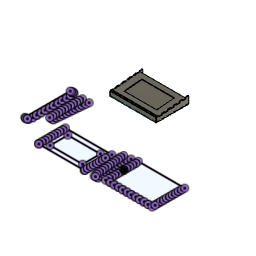
lazerskurður v8 (Autodesk Fusion 360 design; units mm, degrees)
Autodesk Fusion 360 part; units mm, degrees
sketch "Sketch1" plane through (0, 0, 0) normal (0, 0, 1) x (1, 0, 0)
  line L0 (0, 0) -> (314, 0)
  line L1 (314, 0) -> (314, 220)
  line L2 (314, 220) -> (0, 220)
  line L3 (0, 220) -> (0, 0)
  dimension "d8" = 314
  dimension "d9" = 220
  constraint horizontal L0
  constraint vertical L1
  constraint horizontal L2
  constraint vertical L3
  constraint coincident L0.start L3.end
  measures "d8" distance of L0.start L0.end
  measures "d9" distance of L0.start L2.end
extrude "Extrude1" add sketch "Sketch1" along normal blind 4 makes body 1
sketch "Sketch2" plane through (0, 0, 0) normal (0, -1, 0) x (1, 0, 0)
  line L0 (0, 0) -> (314, 0)
  line L1 (314, 0) -> (314, 4)
  line L2 (314, 4) -> (0, 4)
  line L3 (0, 4) -> (0, 0)
sketch "Sketch3" plane through (0, 0, 0) normal (-1, 0, 0) x (0, -1, 0)
  line L0 (-220, 0) -> (0, 0)
  line L1 (0, 0) -> (0, 4)
  line L2 (0, 4) -> (-220, 4)
  line L3 (-220, 4) -> (-220, 0)
  line L4 (-200, 0) -> (-180, 0)
  line L5 (-180, 0) -> (-180, 4)
  line L6 (-180, 4) -> (-200, 4)
  line L7 (-200, 4) -> (-200, 0)
  dimension "d12" = 20
  dimension "d13" = 20
  constraint horizontal L4
  constraint vertical L5
  constraint horizontal L6
  constraint vertical L7
  constraint coincident L2 L5.end
  constraint coincident L0 L4.start
  measures "d12" distance of L5.end L6.end
  measures "d13" distance of L3 L7
extrude "Extrude2" cut sketch "Sketch3" against normal blind 4 contours L0 L2 L4 L5 L6 L7 bodies 1
pattern_linear "R-Pattern1" count 5 spacing 40 along (0, -1, 0) of "Extrude2"
sketch "Sketch4" plane through (0, 0, 0) normal (1, 0, 0) x (0, 1, 0)
  line L0 (220, 0) -> (220, 50)
  line L1 (0, 0) -> (0, 30)
  line L2 (0, 30) -> (220, 50)
  line L3 (0, 30) -> (0, 0)
  line L4 (220, 0) -> (0, 0)
  dimension "d20" = 50
  dimension "d21" = 30
  constraint vertical L0
  constraint coincident L1.start L3.end
  constraint vertical L1
  constraint perpendicular L3 L4
  measures "d20" distance of L0.start L0.end
  measures "d21" distance of L1.start L1.end
extrude "Extrude3" add sketch "Sketch4" along normal blind 4 separate body makes body 2
combine "Combine1" operation cut target body 2 tool bodies 1 keep tools
sketch "Sketch5" plane through (0, -2.7049, 29.7541) normal (0, -0.090536, 0.995893) x (1, 0, 0)
  line L0 (0, 223.6233) -> (0, 2.7161)
  line L1 (0, 2.7161) -> (4, 2.7161)
  line L2 (4, 2.7161) -> (4, 223.6233)
  line L3 (4, 223.6233) -> (0, 223.6233)
  line L4 (0, 203.5408) -> (4, 203.5408)
  line L5 (4, 203.5408) -> (4, 183.4583)
  line L6 (4, 183.4583) -> (0, 183.4583)
  line L7 (0, 183.4583) -> (0, 203.5408)
  dimension "d27" = 20.0825
  dimension "d28" = 20.0825
  constraint horizontal L4
  constraint vertical L5
  constraint horizontal L6
  constraint vertical L7
  constraint coincident L2 L5.end
  constraint coincident L0 L4.start
  measures "d27" distance of L4.start L6.end
  measures "d28" distance of L3 L4
extrude "Extrude4" cut sketch "Sketch5" against normal blind 8 contours L0 L2 L4 L5 L6 L7 bodies 2
pattern_linear "R-Pattern2" count 5 spacing 40.1649 along (0, -0.995893, -0.090536) of "Extrude4"
sketch "Sketch6" plane through (0, -1.9806, 21.787) normal (0, -0.090536, 0.995893) x (1, 0, 0)
  line L0 (0, 183.4583) -> (4, 183.4583)
  line L1 (4, 183.4583) -> (4, 203.5408)
  line L2 (4, 203.5408) -> (0, 203.5408)
  line L3 (0, 203.5408) -> (0, 183.4583)
  line L4 (0, 220) -> (310, 220)
  line L5 (310, 220) -> (310, 0)
  line L6 (310, 0) -> (0, 0)
  line L7 (0, 220) -> (0, 0)
  constraint perpendicular L1 L4
  constraint perpendicular L2 L5
  constraint coincident L6.end L7.end
  constraint perpendicular L5 L6
  constraint perpendicular L6 L7
combine "Combine2" operation cut target body 1 tool bodies 2 keep tools
sketch "Sketch7" plane through (0, 0, 0) normal (0, -1, 0) x (1, 0, 0)
  line L0 (28.5455, 4) -> (57.0909, 4)
  line L1 (57.0909, 4) -> (57.0909, 0)
  line L2 (57.0909, 0) -> (28.5455, 0)
  line L3 (28.5455, 0) -> (28.5455, 4)
  line L4 (0, 4) -> (0, 0)
  dimension "d42" = 28.5455
  dimension "d43" = 28.5455
  constraint horizontal L0
  constraint vertical L1
  constraint horizontal L2
  constraint vertical L3
  measures "d42" distance of L0.start L0.end
  measures "d43" distance of L3 L4
extrude "Extrude7" cut sketch "Sketch7" against normal blind 4 bodies 1
pattern_linear "R-Pattern3" count 5 spacing 57.0909 along (1, 0, 0) of "Extrude7"
sketch "Sketch11" plane through (0, 0, 0) normal (0, -1, 0) x (1, 0, 0)
  line L0 (0, 4) -> (4, 4)
  line L1 (4, 4) -> (4, 30)
  line L2 (4, 30) -> (0, 30)
  line L3 (0, 30) -> (0, 4)
  line L4 (0, 12.6667) -> (4, 12.6667)
  line L5 (4, 12.6667) -> (4, 21.3333)
  line L6 (4, 21.3333) -> (0, 21.3333)
  line L7 (0, 21.3333) -> (0, 12.6667)
  dimension "d56" = 8.6667
  dimension "d57" = 8.6667
  constraint horizontal L4
  constraint vertical L5
  constraint horizontal L6
  constraint vertical L7
  constraint coincident L1 L5.end
  constraint coincident L3 L4.start
  measures "d56" distance of L4.start L6.end
  measures "d57" distance of L0 L4
extrude "Extrude8" cut sketch "Sketch11" against normal blind 4 contours L1 L3 L4 L5 L6 L7 bodies 2
extrude "Extrude9" add 1 faces at (4, 213.5748, 31.4049) along direction (-1, 0, 0) blind 4 from surface at -310 separate body on bodies 2 makes body 3
combine "Combine6" operation cut target body 1 tool bodies 3 keep tools
sketch "Sketch12" plane through (0, 0, 0) normal (0, -1, 0) x (1, 0, 0)
  line L0 (0, 0) -> (0, 30)
  line L1 (0, 30) -> (310, 30)
  line L2 (310, 30) -> (310, 0)
  line L3 (310, 0) -> (0, 0)
  constraint coincident L0.start L3.end
  constraint vertical L0
  constraint perpendicular L0 L1
  constraint perpendicular L1 L2
  constraint perpendicular L0 L3
sketch "Sketch13" plane through (0, -2.3428, 25.7705) normal (0, -0.090536, 0.995893) x (1, 0, 0)
  line L0 (310, 0) -> (310, 220)
  line L1 (310, 220) -> (4, 220)
  line L2 (4, 220) -> (4, 203.5408)
  line L3 (4, 203.5408) -> (0, 203.5408)
  line L4 (0, 2.3524) -> (0, 0)
  line L5 (0, 183.4583) -> (4, 183.4583)
  line L6 (4, 183.4583) -> (4, 163.3759)
  line L7 (4, 163.3759) -> (0, 163.3759)
  line L8 (0, 163.3759) -> (0, 143.2934)
  line L9 (0, 143.2934) -> (4, 143.2934)
  line L10 (4, 143.2934) -> (4, 123.2109)
  line L11 (4, 123.2109) -> (0, 123.2109)
  line L12 (0, 123.2109) -> (0, 103.1284)
  line L13 (0, 103.1284) -> (4, 103.1284)
  line L14 (4, 103.1284) -> (4, 83.046)
  line L15 (4, 83.046) -> (0, 83.046)
  line L16 (0, 83.046) -> (0, 62.9635)
  line L17 (0, 62.9635) -> (4, 62.9635)
  line L18 (4, 62.9635) -> (4, 42.881)
  line L19 (4, 42.881) -> (0, 42.881)
  line L20 (0, 42.881) -> (0, 22.7985)
  line L21 (0, 22.7985) -> (4, 22.7985)
  line L22 (4, 22.7985) -> (4, 2.3524)
  line L23 (50, 190) -> (270, 190)
  line L24 (270, 190) -> (270, 40)
  line L25 (270, 40) -> (50, 40)
  line L26 (50, 40) -> (50, 190)
  line L27 (4, 2.3524) -> (0, 2.3524)
  line L28 (0, 0) -> (310, 0)
  line L29 (0, 203.5408) -> (0, 183.4583)
  constraint horizontal L23
  constraint vertical L24
  constraint horizontal L25
  constraint vertical L26
sketch "Sketch16" plane through (0, -1.9806, 21.787) normal (0, -0.090536, 0.995893) x (1, 0, 0)
  line L0 (0, 183.4583) -> (4, 183.4583)
  line L1 (4, 183.4583) -> (4, 203.5408)
  line L2 (4, 203.5408) -> (0, 203.5408)
  line L3 (0, 203.5408) -> (0, 183.4583)
  line L4 (0, 203.5408) -> (313.7054, 203.5408)
  line L5 (313.7054, 203.5408) -> (313.7054, 20)
  line L6 (313.7054, 20) -> (0, 20)
  line L7 (0, 20) -> (0, 203.5408)
  constraint coincident L2.end L3.start
  constraint perpendicular L3 L4
  constraint perpendicular L4 L5
  constraint perpendicular L5 L6
  constraint perpendicular L6 L7
extrude "Extrude13" add sketch "Sketch16" along normal blind 4 separate body makes body 4
combine "Combine10" operation cut target body 4 tool bodies 2 keep tools
combine "Combine11" operation cut target body 4 tool bodies 3 keep tools
sketch "Sketch17" plane through (0, 0, 0) normal (0, -1, 0) x (1, 0, 0)
  line L0 (4, 12.6667) -> (0, 12.6667)
  line L1 (0, 12.6667) -> (0, 4)
  line L2 (0, 4) -> (4, 4)
  line L3 (4, 4) -> (4, 12.6667)
  line L4 (0, 0) -> (314, 0)
  line L5 (314, 0) -> (314, 30)
  line L6 (314, 30) -> (0, 30)
  line L7 (0, 30) -> (0, 0)
  constraint horizontal L4
  constraint vertical L5
  constraint horizontal L6
  constraint vertical L7
  constraint coincident L4.start L7.end
extrude "Extrude14" add sketch "Sketch17" against normal blind 4 separate body contours L0 L2 L3 L4 L5 L6 L7 makes body 5
combine "Combine12" operation cut target body 5 tool bodies 3 keep tools
combine "Combine13" operation cut target body 5 tool bodies 2 keep tools
combine "Combine14" operation cut target body 5 tool bodies 1 keep tools
sketch "Sketch18" plane through (0, -2.3428, 25.7705) normal (0, -0.090536, 0.995893) x (1, 0, 0)
  line L0 (310, 183.4583) -> (313.7054, 183.4583)
  line L1 (313.7054, 183.4583) -> (313.7054, 203.5408)
  line L2 (313.7054, 203.5408) -> (0, 203.5408)
  line L3 (0, 203.5408) -> (0, 183.4583)
  line L4 (0, 183.4583) -> (4, 183.4583)
  line L5 (4, 183.4583) -> (4, 163.3759)
  line L6 (4, 163.3759) -> (0, 163.3759)
  line L7 (0, 163.3759) -> (0, 143.2934)
  line L8 (0, 143.2934) -> (4, 143.2934)
  line L9 (4, 143.2934) -> (4, 123.2109)
  line L10 (4, 123.2109) -> (0, 123.2109)
  line L11 (0, 123.2109) -> (0, 103.1284)
  line L12 (0, 103.1284) -> (4, 103.1284)
  line L13 (4, 103.1284) -> (4, 83.046)
  line L14 (4, 83.046) -> (0, 83.046)
  line L15 (0, 83.046) -> (0, 62.9635)
  line L16 (0, 62.9635) -> (4, 62.9635)
  line L17 (4, 62.9635) -> (4, 42.881)
  line L18 (4, 42.881) -> (0, 42.881)
  line L19 (0, 42.881) -> (0, 22.7985)
  line L20 (0, 22.7985) -> (4, 22.7985)
  line L21 (4, 22.7985) -> (4, 20)
  line L22 (4, 20) -> (310, 20)
  line L23 (310, 20) -> (310, 22.7985)
  line L24 (310, 22.7985) -> (313.7054, 22.7985)
  line L25 (313.7054, 22.7985) -> (313.7054, 42.881)
  line L26 (313.7054, 42.881) -> (310, 42.881)
  line L27 (310, 42.881) -> (310, 62.9635)
  line L28 (310, 62.9635) -> (313.7054, 62.9635)
  line L29 (313.7054, 62.9635) -> (313.7054, 83.046)
  line L30 (313.7054, 83.046) -> (310, 83.046)
  line L31 (310, 83.046) -> (310, 103.1284)
  line L32 (310, 103.1284) -> (313.7054, 103.1284)
  line L33 (313.7054, 103.1284) -> (313.7054, 123.2109)
  line L34 (313.7054, 123.2109) -> (310, 123.2109)
  line L35 (310, 123.2109) -> (310, 143.2934)
  line L36 (310, 143.2934) -> (313.7054, 143.2934)
  line L37 (313.7054, 143.2934) -> (313.7054, 163.3759)
  line L38 (313.7054, 163.3759) -> (310, 163.3759)
  line L39 (310, 163.3759) -> (310, 183.4583)
  line L40 (50, 170) -> (270, 170)
  line L41 (270, 170) -> (270, 50)
  line L42 (270, 50) -> (50, 50)
  line L43 (50, 50) -> (50, 170)
  dimension "d81" = 220
  dimension "d82" = 120
  constraint horizontal L40
  constraint vertical L41
  constraint horizontal L42
  constraint vertical L43
  measures "d81" distance of L40.start L40.end
  measures "d82" distance of L40.end L41.end
extrude "Extrude15" cut sketch "Sketch18" against normal blind 4 contours L40 L41 L42 L43 bodies 4
copy_body "CopyPasteBodies1" bodies 2 1 3 4 5 makes body 6 makes body 7 makes body 8 makes body 9 makes body 10
move_body "Move1" bodies 6 7 8 9 10 to x (1, 0, 0) y (0, 1, 0) z (0, 0, 1) at (89.2119, -176.0551, -86.8432)
move_body "Move2" bodies 6 to x (0, 0, -1) y (0, 1, 0) z (1, 0, 0) at (98.3429, 35.2103, -32.1331)
move_body "Move3" bodies 9 to x (1, 0, 0) y (0, 0.996195, -0.087156) z (0, 0.087156, 0.996195) at (39.57, -152.6482, -122.2608)
move_body "Move4" bodies 9 to x (1, 0, 0) y (0, 1, 0) z (0, 0, 1) at (0, -16.2423, 45.5832)
move_body "Move5" bodies 10 to x (0, 1, 0) y (0, 0, -1) z (-1, 0, 0) at (95.3934, -119.6113, -495.9946)
move_body "Move6" bodies 8 to x (0, 0.090536, -0.995893) y (-0.090536, 0.991803, 0.090164) z (0.995893, 0.090164, 0.008197) at (447.8824, -31.7365, 349.1019)
move_body "Move7" bodies 8 to x (1, 0, 0) y (0, 1, 0) z (0, 0, 1) at (27.4998, -31.7778, -4.278)
move_body "Move8" bodies 10 to x (1, 0, 0) y (0, 1, 0) z (0, 0, 1) at (-82.2593, 0, 198.051)
move_body "Move9" bodies 8 to x (0.999969, -0.000373, 0.007889) y (0.001056, 0.996226, -0.086795) z (-0.007827, 0.086801, 0.996195) at (-0.3498, 4.8832, -11.2116)
sketch "Sketch19" plane through (0, 0, -82.8432) normal (0, 0, 1) x (-1, 0, 0)
  line L0 (-399.2119, 156.0551) -> (-399.2119, 136.0551)
  line L1 (-399.2119, 136.0551) -> (-403.2119, 136.0551)
  line L2 (-403.2119, 136.0551) -> (-403.2119, 116.0551)
  line L3 (-403.2119, 116.0551) -> (-399.2119, 116.0551)
  line L4 (-399.2119, 116.0551) -> (-399.2119, 96.0551)
  line L5 (-399.2119, 96.0551) -> (-403.2119, 96.0551)
  line L6 (-403.2119, 96.0551) -> (-403.2119, 76.0551)
  line L7 (-403.2119, 76.0551) -> (-399.2119, 76.0551)
  line L8 (-399.2119, 76.0551) -> (-399.2119, 56.0551)
  line L9 (-399.2119, 56.0551) -> (-403.2119, 56.0551)
  line L10 (-403.2119, 56.0551) -> (-403.2119, 36.0551)
  line L11 (-403.2119, 36.0551) -> (-399.2119, 36.0551)
  line L12 (-399.2119, 36.0551) -> (-399.2119, 16.0551)
  line L13 (-399.2119, 16.0551) -> (-403.2119, 16.0551)
  line L14 (-403.2119, 16.0551) -> (-403.2119, -3.9449)
  line L15 (-403.2119, -3.9449) -> (-399.2119, -3.9449)
  line L16 (-399.2119, -3.9449) -> (-399.2119, -23.9449)
  line L17 (-399.2119, -23.9449) -> (-403.2119, -23.9449)
  line L18 (-403.2119, -23.9449) -> (-403.2119, -43.9449)
  line L19 (-403.2119, -43.9449) -> (-89.2119, -43.9449)
  line L20 (-89.2119, -43.9449) -> (-89.2119, -23.9449)
  line L21 (-89.2119, -23.9449) -> (-93.2119, -23.9449)
  line L22 (-93.2119, -23.9449) -> (-93.2119, -3.9449)
  line L23 (-93.2119, -3.9449) -> (-89.2119, -3.9449)
  line L24 (-89.2119, -3.9449) -> (-89.2119, 16.0551)
  line L25 (-89.2119, 16.0551) -> (-93.2119, 16.0551)
  line L26 (-93.2119, 16.0551) -> (-93.2119, 36.0551)
  line L27 (-93.2119, 36.0551) -> (-89.2119, 36.0551)
  line L28 (-89.2119, 36.0551) -> (-89.2119, 56.0551)
  line L29 (-89.2119, 56.0551) -> (-93.2119, 56.0551)
  line L30 (-93.2119, 56.0551) -> (-93.2119, 76.0551)
  line L31 (-93.2119, 76.0551) -> (-89.2119, 76.0551)
  line L32 (-89.2119, 76.0551) -> (-89.2119, 96.0551)
  line L33 (-89.2119, 96.0551) -> (-93.2119, 96.0551)
  line L34 (-93.2119, 96.0551) -> (-93.2119, 116.0551)
  line L35 (-93.2119, 116.0551) -> (-89.2119, 116.0551)
  line L36 (-89.2119, 116.0551) -> (-89.2119, 136.0551)
  line L37 (-89.2119, 136.0551) -> (-93.2119, 136.0551)
  line L38 (-93.2119, 136.0551) -> (-93.2119, 156.0551)
  line L39 (-93.2119, 156.0551) -> (-89.2119, 156.0551)
  line L40 (-89.2119, 156.0551) -> (-89.2119, 176.0551)
  line L41 (-89.2119, 176.0551) -> (-117.7574, 176.0551)
  line L42 (-117.7574, 176.0551) -> (-117.7574, 172.0551)
  line L43 (-117.7574, 172.0551) -> (-146.3028, 172.0551)
  line L44 (-146.3028, 172.0551) -> (-146.3028, 176.0551)
  line L45 (-146.3028, 176.0551) -> (-174.8483, 176.0551)
  line L46 (-174.8483, 176.0551) -> (-174.8483, 172.0551)
  line L47 (-174.8483, 172.0551) -> (-203.3938, 172.0551)
  line L48 (-203.3938, 172.0551) -> (-203.3938, 176.0551)
  line L49 (-203.3938, 176.0551) -> (-231.9392, 176.0551)
  line L50 (-231.9392, 176.0551) -> (-231.9392, 172.0551)
  line L51 (-231.9392, 172.0551) -> (-260.4847, 172.0551)
  line L52 (-260.4847, 172.0551) -> (-260.4847, 176.0551)
  line L53 (-260.4847, 176.0551) -> (-289.0301, 176.0551)
  line L54 (-289.0301, 176.0551) -> (-289.0301, 172.0551)
  line L55 (-289.0301, 172.0551) -> (-317.5756, 172.0551)
  line L56 (-317.5756, 172.0551) -> (-317.5756, 176.0551)
  line L57 (-317.5756, 176.0551) -> (-346.121, 176.0551)
  line L58 (-346.121, 176.0551) -> (-346.121, 172.0551)
  line L59 (-346.121, 172.0551) -> (-374.6665, 172.0551)
  line L60 (-374.6665, 172.0551) -> (-374.6665, 176.0551)
  line L61 (-374.6665, 176.0551) -> (-403.2119, 176.0551)
  line L62 (-403.2119, 176.0551) -> (-403.2119, 156.0551)
  line L63 (-403.2119, 156.0551) -> (-399.2119, 156.0551)
sketch "Sketch20" plane through (0, 0, -82.8432) normal (0, 0, 1) x (-1, 0, 0)
move_body "Move10" bodies 9 6 to x (1, 0, 0) y (0, 1, 0) z (0, 0, 1) at (-174.0822, -104.8957, 0)
move_body "Move11" bodies 8 to x (1, 0, 0) y (0, 1, 0) z (0, 0, 1) at (-76.6506, -226.9909, -24.5255)
move_body "Move12" bodies 7 to x (1, 0, 0) y (0, 1, 0) z (0, 0, 1) at (305.7598, -246.2445, 0)
move_body "Move13" bodies 10 to x (1, 0, 0) y (0, 1, 0) z (0, 0, 1) at (-314.456, -301.2845, 0)
sketch "Sketch21" plane through (0, 0, -82.8432) normal (0, 0, 1) x (1, 0, 0)
  line L0 (-218.4787, -327.6839) -> (-218.4787, -303.1384)
  line L1 (-218.4787, -303.1384) -> (-214.4787, -303.1384)
  line L2 (-214.4787, -303.1384) -> (-214.4787, -274.5929)
  line L3 (-214.4787, -274.5929) -> (-218.4787, -274.5929)
  line L4 (-218.4787, -274.5929) -> (-218.4787, -246.0475)
  line L5 (-218.4787, -246.0475) -> (-214.4787, -246.0475)
  line L6 (-214.4787, -246.0475) -> (-214.4787, -217.502)
  line L7 (-214.4787, -217.502) -> (-218.4787, -217.502)
  line L8 (-218.4787, -217.502) -> (-218.4787, -188.9566)
  line L9 (-218.4787, -188.9566) -> (-214.4787, -188.9566)
  line L10 (-214.4787, -188.9566) -> (-214.4787, -160.4111)
  line L11 (-214.4787, -160.4111) -> (-218.4787, -160.4111)
  line L12 (-218.4787, -160.4111) -> (-218.4787, -131.8657)
  line L13 (-218.4787, -131.8657) -> (-214.4787, -131.8657)
  line L14 (-214.4787, -131.8657) -> (-214.4787, -103.3202)
  line L15 (-214.4787, -103.3202) -> (-218.4787, -103.3202)
  line L16 (-218.4787, -103.3202) -> (-218.4787, -74.7748)
  line L17 (-218.4787, -74.7748) -> (-214.4787, -74.7748)
  line L18 (-214.4787, -74.7748) -> (-214.4787, -46.2293)
  line L19 (-214.4787, -46.2293) -> (-218.4787, -46.2293)
  line L20 (-218.4787, -46.2293) -> (-218.4787, -21.6839)
  line L21 (-218.4787, -21.6839) -> (-227.1454, -21.6839)
  line L22 (-227.1454, -21.6839) -> (-227.1454, -17.6839)
  line L23 (-227.1454, -17.6839) -> (-235.812, -17.6838)
  line L24 (-235.812, -17.6838) -> (-235.812, -21.6839)
  line L25 (-235.812, -21.6839) -> (-244.4787, -21.6839)
  line L26 (-244.4787, -21.6839) -> (-244.4787, -327.6839)
  line L27 (-244.4787, -327.6839) -> (-235.812, -327.6839)
  line L28 (-235.812, -327.6839) -> (-235.812, -331.6839)
  line L29 (-235.812, -331.6839) -> (-227.1454, -331.6839)
  line L30 (-227.1454, -331.6839) -> (-227.1454, -327.6839)
  line L31 (-227.1454, -327.6839) -> (-218.4787, -327.6839)
  line L32 (-149.9158, -245.7405) -> (-149.9158, -241.7405)
  line L33 (-149.9158, -241.7405) -> (-141.2491, -241.7405)
  line L34 (-141.2491, -241.7405) -> (-141.2491, -245.7405)
  line L35 (-141.2491, -245.7405) -> (-132.5825, -245.7405)
  line L36 (-132.5825, -245.7405) -> (-130.7643, -225.7405)
  line L37 (-130.7643, -225.7405) -> (-138.7314, -225.0162)
  line L38 (-138.7314, -225.0162) -> (-136.9133, -205.0162)
  line L39 (-136.9133, -205.0162) -> (-128.9461, -205.7405)
  line L40 (-128.9461, -205.7405) -> (-127.1279, -185.7405)
  line L41 (-127.1279, -185.7405) -> (-135.0951, -185.0162)
  line L42 (-135.0951, -185.0162) -> (-133.2769, -165.0162)
  line L43 (-133.2769, -165.0162) -> (-125.3097, -165.7405)
  line L44 (-125.3097, -165.7405) -> (-123.4916, -145.7405)
  line L45 (-123.4916, -145.7405) -> (-131.4587, -145.0162)
  line L46 (-131.4587, -145.0162) -> (-129.6405, -125.0162)
  line L47 (-129.6405, -125.0162) -> (-121.6734, -125.7405)
  line L48 (-121.6734, -125.7405) -> (-119.8552, -105.7405)
  line L49 (-119.8552, -105.7405) -> (-127.8223, -105.0162)
  line L50 (-127.8223, -105.0162) -> (-126.0042, -85.0162)
  line L51 (-126.0042, -85.0162) -> (-118.037, -85.7405)
  line L52 (-118.037, -85.7405) -> (-116.2188, -65.7405)
  line L53 (-116.2188, -65.7405) -> (-124.186, -65.0162)
  line L54 (-124.186, -65.0162) -> (-122.3678, -45.0162)
  line L55 (-122.3678, -45.0162) -> (-114.4007, -45.7405)
  line L56 (-114.4007, -45.7405) -> (-112.5825, -25.7405)
  line L57 (-112.5825, -25.7405) -> (-158.5825, -25.7405)
  line L58 (-158.5825, -25.7405) -> (-158.5825, -45.7405)
  line L59 (-158.5825, -45.7405) -> (-162.5825, -45.7405)
  line L60 (-162.5825, -45.7405) -> (-162.5825, -65.7405)
  line L61 (-162.5825, -65.7405) -> (-158.5825, -65.7405)
  line L62 (-158.5825, -65.7405) -> (-158.5825, -85.7405)
  line L63 (-158.5825, -85.7405) -> (-162.5825, -85.7405)
  line L64 (-162.5825, -85.7405) -> (-162.5825, -105.7405)
  line L65 (-162.5825, -105.7405) -> (-158.5825, -105.7405)
  line L66 (-158.5825, -105.7405) -> (-158.5825, -125.7405)
  line L67 (-158.5825, -125.7405) -> (-162.5825, -125.7405)
  line L68 (-162.5825, -125.7405) -> (-162.5825, -145.7405)
  line L69 (-162.5825, -145.7405) -> (-158.5825, -145.7405)
  line L70 (-158.5825, -145.7405) -> (-158.5825, -165.7405)
  line L71 (-158.5825, -165.7405) -> (-162.5825, -165.7405)
  line L72 (-162.5825, -165.7405) -> (-162.5825, -185.7405)
  line L73 (-162.5825, -185.7405) -> (-158.5825, -185.7405)
  line L74 (-158.5825, -185.7405) -> (-158.5825, -205.7405)
  line L75 (-158.5825, -205.7405) -> (-162.5825, -205.7405)
  line L76 (-162.5825, -205.7405) -> (-162.5825, -225.7405)
  line L77 (-162.5825, -225.7405) -> (-158.5825, -225.7405)
  line L78 (-158.5825, -225.7405) -> (-158.5825, -245.7405)
  line L79 (-158.5825, -245.7405) -> (-149.9158, -245.7405)
  line L80 (224.6997, -286.829) -> (224.6997, -406.8283)
  line L81 (224.6997, -406.8283) -> (4.6997, -406.8283)
  line L82 (4.6997, -406.8283) -> (4.6997, -286.829)
  line L83 (4.6997, -286.829) -> (224.6997, -286.829)
  line L84 (264.6997, -273.3707) -> (268.4052, -273.3707)
  line L85 (268.4052, -273.3707) -> (268.4052, -253.2884)
  line L86 (268.4052, -253.2884) -> (-45.3003, -253.2884)
  line L87 (-45.3003, -253.2884) -> (-45.3003, -273.3707)
  line L88 (-45.3003, -273.3707) -> (-41.3003, -273.3707)
  line L89 (-41.3003, -273.3707) -> (-41.3003, -293.4531)
  line L90 (-41.3003, -293.4531) -> (-45.3003, -293.4531)
  line L91 (-45.3003, -293.4531) -> (-45.3003, -313.5354)
  line L92 (-45.3003, -313.5354) -> (-41.3003, -313.5354)
  line L93 (-41.3003, -313.5354) -> (-41.3003, -333.6178)
  line L94 (-41.3003, -333.6178) -> (-45.3003, -333.6178)
  line L95 (-45.3003, -333.6178) -> (-45.3003, -353.7002)
  line L96 (-45.3003, -353.7002) -> (-41.3003, -353.7002)
  line L97 (-41.3003, -353.7002) -> (-41.3003, -373.7825)
  line L98 (-41.3003, -373.7825) -> (-45.3003, -373.7825)
  line L99 (-45.3003, -373.7825) -> (-45.3003, -393.8649)
  line L100 (-45.3003, -393.8649) -> (-41.3003, -393.8649)
  line L101 (-41.3003, -393.8649) -> (-41.3003, -413.9472)
  line L102 (-41.3003, -413.9472) -> (-45.3003, -413.9472)
  line L103 (-45.3003, -413.9472) -> (-45.3003, -434.0296)
  line L104 (-45.3003, -434.0296) -> (-41.3003, -434.0296)
  line L105 (-41.3003, -434.0296) -> (-41.3003, -436.8281)
  line L106 (-41.3003, -436.8281) -> (264.6997, -436.8281)
  line L107 (264.6997, -436.8281) -> (264.6997, -434.0296)
  line L108 (264.6997, -434.0296) -> (268.4052, -434.0296)
  line L109 (268.4052, -434.0296) -> (268.4052, -413.9472)
  line L110 (268.4052, -413.9472) -> (264.6997, -413.9472)
  line L111 (264.6997, -413.9472) -> (264.6997, -393.8649)
  line L112 (264.6997, -393.8649) -> (268.4052, -393.8649)
  line L113 (268.4052, -393.8649) -> (268.4052, -373.7825)
  line L114 (268.4052, -373.7825) -> (264.6997, -373.7825)
  line L115 (264.6997, -373.7825) -> (264.6997, -353.7002)
  line L116 (264.6997, -353.7002) -> (268.4052, -353.7002)
  line L117 (268.4052, -353.7002) -> (268.4052, -333.6178)
  line L118 (268.4052, -333.6178) -> (264.6997, -333.6178)
  line L119 (264.6997, -333.6178) -> (264.6997, -313.5354)
  line L120 (264.6997, -313.5354) -> (268.4052, -313.5354)
  line L121 (268.4052, -313.5354) -> (268.4052, -293.4531)
  line L122 (268.4052, -293.4531) -> (264.6997, -293.4531)
  line L123 (264.6997, -293.4531) -> (264.6997, -273.3707)
  line L124 (340.3969, -432.1727) -> (349.028, -431.3912)
  line L125 (349.028, -431.3912) -> (349.3887, -435.3749)
  line L126 (349.3887, -435.3749) -> (358.0198, -434.5935)
  line L127 (358.0198, -434.5935) -> (358.0267, -414.5112)
  line L128 (358.0267, -414.5112) -> (350.0269, -414.5082)
  line L129 (350.0269, -414.5082) -> (350.0338, -394.4258)
  line L130 (350.0338, -394.4258) -> (358.0336, -394.4288)
  line L131 (358.0336, -394.4288) -> (358.0405, -374.3465)
  line L132 (358.0405, -374.3465) -> (350.0407, -374.3435)
  line L133 (350.0407, -374.3435) -> (350.0476, -354.2612)
  line L134 (350.0476, -354.2612) -> (358.0474, -354.2642)
  line L135 (358.0474, -354.2642) -> (358.0543, -334.1818)
  line L136 (358.0543, -334.1818) -> (350.0545, -334.1788)
  line L137 (350.0545, -334.1788) -> (350.0614, -314.0965)
  line L138 (350.0614, -314.0965) -> (358.0611, -314.0995)
  line L139 (358.0611, -314.0995) -> (358.068, -294.0172)
  line L140 (358.068, -294.0172) -> (350.0683, -294.0142)
  line L141 (350.0683, -294.0142) -> (350.0752, -273.9319)
  line L142 (350.0752, -273.9319) -> (358.0749, -273.9348)
  line L143 (358.0749, -273.9348) -> (358.0818, -253.8525)
  line L144 (358.0818, -253.8525) -> (350.0821, -253.8495)
  line L145 (350.0821, -253.8495) -> (350.089, -233.7672)
  line L146 (350.089, -233.7672) -> (358.0887, -233.7702)
  line L147 (358.0887, -233.7702) -> (358.0956, -213.6878)
  line L148 (358.0956, -213.6878) -> (312.2845, -217.8354)
  line L149 (312.2845, -217.8354) -> (314.0883, -237.7538)
  line L150 (314.0883, -237.7538) -> (310.1048, -238.1144)
  line L151 (310.1048, -238.1144) -> (311.9086, -258.0328)
  line L152 (311.9086, -258.0328) -> (315.8922, -257.6722)
  line L153 (315.8922, -257.6722) -> (317.696, -277.5906)
  line L154 (317.696, -277.5906) -> (313.7124, -277.9512)
  line L155 (313.7124, -277.9512) -> (315.5162, -297.8696)
  line L156 (315.5162, -297.8696) -> (319.4998, -297.509)
  line L157 (319.4998, -297.509) -> (321.3036, -317.4274)
  line L158 (321.3036, -317.4274) -> (317.3201, -317.788)
  line L159 (317.3201, -317.788) -> (319.1239, -337.7064)
  line L160 (319.1239, -337.7064) -> (323.1075, -337.3458)
  line L161 (323.1075, -337.3458) -> (324.9113, -357.2642)
  line L162 (324.9113, -357.2642) -> (320.9277, -357.6248)
  line L163 (320.9277, -357.6248) -> (322.7315, -377.5432)
  line L164 (322.7315, -377.5432) -> (326.7151, -377.1826)
  line L165 (326.7151, -377.1826) -> (328.5189, -397.101)
  line L166 (328.5189, -397.101) -> (324.5354, -397.4616)
  line L167 (324.5354, -397.4616) -> (326.3392, -417.38)
  line L168 (326.3392, -417.38) -> (330.3228, -417.0194)
  line L169 (330.3228, -417.0194) -> (332.1266, -436.9378)
  line L170 (332.1266, -436.9378) -> (340.7577, -436.1563)
  line L171 (340.7577, -436.1563) -> (340.3969, -432.1727)
  line L172 (704.9717, -402.2996) -> (704.9717, -382.2996)
  line L173 (704.9717, -382.2996) -> (708.9717, -382.2996)
  line L174 (708.9717, -382.2996) -> (708.9717, -362.2996)
  line L175 (708.9717, -362.2996) -> (704.9717, -362.2996)
  line L176 (704.9717, -362.2996) -> (704.9717, -342.2996)
  line L177 (704.9717, -342.2996) -> (708.9717, -342.2996)
  line L178 (708.9717, -342.2996) -> (708.9717, -322.2996)
  line L179 (708.9717, -322.2996) -> (704.9717, -322.2996)
  line L180 (704.9717, -322.2996) -> (704.9717, -302.2996)
  line L181 (704.9717, -302.2996) -> (708.9717, -302.2996)
  line L182 (708.9717, -302.2996) -> (708.9717, -282.2996)
  line L183 (708.9717, -282.2996) -> (704.9717, -282.2996)
  line L184 (704.9717, -282.2996) -> (704.9717, -262.2996)
  line L185 (704.9717, -262.2996) -> (708.9717, -262.2996)
  line L186 (708.9717, -262.2996) -> (708.9717, -242.2996)
  line L187 (708.9717, -242.2996) -> (704.9717, -242.2996)
  line L188 (704.9717, -242.2996) -> (704.9717, -222.2996)
  line L189 (704.9717, -222.2996) -> (708.9717, -222.2996)
  line L190 (708.9717, -222.2996) -> (708.9717, -202.2996)
  line L191 (708.9717, -202.2996) -> (394.9717, -202.2996)
  line L192 (394.9717, -202.2996) -> (394.9717, -222.2996)
  line L193 (394.9717, -222.2996) -> (398.9717, -222.2996)
  line L194 (398.9717, -222.2996) -> (398.9717, -242.2996)
  line L195 (398.9717, -242.2996) -> (394.9717, -242.2996)
  line L196 (394.9717, -242.2996) -> (394.9717, -262.2996)
  line L197 (394.9717, -262.2996) -> (398.9717, -262.2996)
  line L198 (398.9717, -262.2996) -> (398.9717, -282.2996)
  line L199 (398.9717, -282.2996) -> (394.9717, -282.2996)
  line L200 (394.9717, -282.2996) -> (394.9717, -302.2996)
  line L201 (394.9717, -302.2996) -> (398.9717, -302.2996)
  line L202 (398.9717, -302.2996) -> (398.9717, -322.2996)
  line L203 (398.9717, -322.2996) -> (394.9717, -322.2996)
  line L204 (394.9717, -322.2996) -> (394.9717, -342.2996)
  line L205 (394.9717, -342.2996) -> (398.9717, -342.2996)
  line L206 (398.9717, -342.2996) -> (398.9717, -362.2996)
  line L207 (398.9717, -362.2996) -> (394.9717, -362.2996)
  line L208 (394.9717, -362.2996) -> (394.9717, -382.2996)
  line L209 (394.9717, -382.2996) -> (398.9717, -382.2996)
  line L210 (398.9717, -382.2996) -> (398.9717, -402.2996)
  line L211 (398.9717, -402.2996) -> (394.9717, -402.2996)
  line L212 (394.9717, -402.2996) -> (394.9717, -422.2996)
  line L213 (394.9717, -422.2996) -> (423.5172, -422.2996)
  line L214 (423.5172, -422.2996) -> (423.5172, -418.2996)
  line L215 (423.5172, -418.2996) -> (452.0626, -418.2996)
  line L216 (452.0626, -418.2996) -> (452.0626, -422.2996)
  line L217 (452.0626, -422.2996) -> (480.6081, -422.2996)
  line L218 (480.6081, -422.2996) -> (480.6081, -418.2996)
  line L219 (480.6081, -418.2996) -> (509.1535, -418.2996)
  line L220 (509.1535, -418.2996) -> (509.1535, -422.2996)
  line L221 (509.1535, -422.2996) -> (537.699, -422.2996)
  line L222 (537.699, -422.2996) -> (537.699, -418.2996)
  line L223 (537.699, -418.2996) -> (566.2444, -418.2996)
  line L224 (566.2444, -418.2996) -> (566.2444, -422.2996)
  line L225 (566.2444, -422.2996) -> (594.7899, -422.2996)
  line L226 (594.7899, -422.2996) -> (594.7899, -418.2996)
  line L227 (594.7899, -418.2996) -> (623.3353, -418.2996)
  line L228 (623.3353, -418.2996) -> (623.3353, -422.2996)
  line L229 (623.3353, -422.2996) -> (651.8808, -422.2996)
  line L230 (651.8808, -422.2996) -> (651.8808, -418.2996)
  line L231 (651.8808, -418.2996) -> (680.4263, -418.2996)
  line L232 (680.4263, -418.2996) -> (680.4263, -422.2996)
  line L233 (680.4263, -422.2996) -> (708.9717, -422.2996)
  line L234 (708.9717, -422.2996) -> (708.9717, -402.2996)
  line L235 (708.9717, -402.2996) -> (704.9717, -402.2996)
  line L236 (-162.6825, -45.6405) -> (-162.6825, -65.8405)
  line L237 (-162.6825, -65.8405) -> (-158.6825, -65.8405)
  line L238 (-158.6825, -65.8405) -> (-158.6825, -85.6405)
  line L239 (-158.6825, -85.6405) -> (-162.6825, -85.6405)
  line L240 (-162.6825, -85.6405) -> (-162.6825, -105.8405)
  line L241 (-162.6825, -105.8405) -> (-158.6825, -105.8405)
  line L242 (-158.6825, -105.8405) -> (-158.6825, -125.6405)
  line L243 (-158.6825, -125.6405) -> (-162.6825, -125.6405)
  line L244 (-162.6825, -125.6405) -> (-162.6825, -145.8405)
  line L245 (-162.6825, -145.8405) -> (-158.6825, -145.8405)
  line L246 (-158.6825, -145.8405) -> (-158.6825, -165.6405)
  line L247 (-158.6825, -165.6405) -> (-162.6825, -165.6405)
  line L248 (-162.6825, -165.6405) -> (-162.6825, -185.8405)
  line L249 (-162.6825, -185.8405) -> (-158.6825, -185.8405)
  line L250 (-158.6825, -185.8405) -> (-158.6825, -205.6405)
  line L251 (-158.6825, -205.6405) -> (-162.6825, -205.6405)
  line L252 (-162.6825, -205.6405) -> (-162.6825, -225.8405)
  line L253 (-162.6825, -225.8405) -> (-158.6825, -225.8405)
  line L254 (-158.6825, -225.8405) -> (-158.6825, -245.8405)
  line L255 (-158.6825, -245.8405) -> (-149.8158, -245.8405)
  line L256 (-149.8158, -245.8405) -> (-149.8158, -241.8405)
  line L257 (-149.8158, -241.8405) -> (-141.3491, -241.8405)
  line L258 (-141.3491, -241.8405) -> (-141.3491, -245.8405)
  line L259 (-141.3491, -245.8405) -> (-132.4912, -245.8405)
  line L260 (-132.4912, -245.8405) -> (-130.6556, -225.65)
  line L261 (-130.6556, -225.65) -> (-138.6228, -224.9257)
  line L262 (-138.6228, -224.9257) -> (-136.8227, -205.1248)
  line L263 (-136.8227, -205.1248) -> (-128.8556, -205.8491)
  line L264 (-128.8556, -205.8491) -> (-127.0193, -185.65)
  line L265 (-127.0193, -185.65) -> (-134.9864, -184.9257)
  line L266 (-134.9864, -184.9257) -> (-133.1864, -165.1248)
  line L267 (-133.1864, -165.1248) -> (-125.2192, -165.8491)
  line L268 (-125.2192, -165.8491) -> (-123.3829, -145.65)
  line L269 (-123.3829, -145.65) -> (-131.3501, -144.9257)
  line L270 (-131.3501, -144.9257) -> (-129.55, -125.1248)
  line L271 (-129.55, -125.1248) -> (-121.5828, -125.8491)
  line L272 (-121.5828, -125.8491) -> (-119.7466, -105.65)
  line L273 (-119.7466, -105.65) -> (-127.7137, -104.9257)
  line L274 (-127.7137, -104.9257) -> (-125.9136, -85.1248)
  line L275 (-125.9136, -85.1248) -> (-117.9465, -85.8491)
  line L276 (-117.9465, -85.8491) -> (-116.1102, -65.65)
  line L277 (-116.1102, -65.65) -> (-124.0773, -64.9257)
  line L278 (-124.0773, -64.9257) -> (-122.2773, -45.1248)
  line L279 (-122.2773, -45.1248) -> (-114.3101, -45.8491)
  line L280 (-114.3101, -45.8491) -> (-112.473, -25.6405)
  line L281 (-112.473, -25.6405) -> (-158.6825, -25.6405)
  line L282 (-158.6825, -25.6405) -> (-158.6825, -45.6405)
  line L283 (-158.6825, -45.6405) -> (-162.6825, -45.6405)
  line L284 (268.5052, -373.6825) -> (264.7997, -373.6825)
  line L285 (264.7997, -373.6825) -> (264.7997, -353.8002)
  line L286 (264.7997, -353.8002) -> (268.5052, -353.8002)
  line L287 (268.5052, -353.8002) -> (268.5052, -333.5178)
  line L288 (268.5052, -333.5178) -> (264.7997, -333.5178)
  line L289 (264.7997, -333.5178) -> (264.7997, -313.6354)
  line L290 (264.7997, -313.6354) -> (268.5052, -313.6354)
  line L291 (268.5052, -313.6354) -> (268.5052, -293.3531)
  line L292 (268.5052, -293.3531) -> (264.7997, -293.3531)
  line L293 (264.7997, -293.3531) -> (264.7997, -273.4707)
  line L294 (264.7997, -273.4707) -> (268.5052, -273.4707)
  line L295 (268.5052, -273.4707) -> (268.5052, -253.1884)
  line L296 (268.5052, -253.1884) -> (-45.4003, -253.1884)
  line L297 (-45.4003, -253.1884) -> (-45.4003, -273.4707)
  line L298 (-45.4003, -273.4707) -> (-41.4003, -273.4707)
  line L299 (-41.4003, -273.4707) -> (-41.4003, -293.3531)
  line L300 (-41.4003, -293.3531) -> (-45.4003, -293.3531)
  line L301 (-45.4003, -293.3531) -> (-45.4003, -313.6354)
  line L302 (-45.4003, -313.6354) -> (-41.4003, -313.6354)
  line L303 (-41.4003, -313.6354) -> (-41.4003, -333.5178)
  line L304 (-41.4003, -333.5178) -> (-45.4003, -333.5178)
  line L305 (-45.4003, -333.5178) -> (-45.4003, -353.8002)
  line L306 (-45.4003, -353.8002) -> (-41.4003, -353.8002)
  line L307 (-41.4003, -353.8002) -> (-41.4003, -373.6825)
  line L308 (-41.4003, -373.6825) -> (-45.4003, -373.6825)
  line L309 (-45.4003, -373.6825) -> (-45.4003, -393.9649)
  line L310 (-45.4003, -393.9649) -> (-41.4003, -393.9649)
  line L311 (-41.4003, -393.9649) -> (-41.4003, -413.8472)
  line L312 (-41.4003, -413.8472) -> (-45.4003, -413.8472)
  line L313 (-45.4003, -413.8472) -> (-45.4003, -434.1296)
  line L314 (-45.4003, -434.1296) -> (-41.4003, -434.1296)
  line L315 (-41.4003, -434.1296) -> (-41.4003, -436.9281)
  line L316 (-41.4003, -436.9281) -> (264.7997, -436.9281)
  line L317 (264.7997, -436.9281) -> (264.7997, -434.1296)
  line L318 (264.7997, -434.1296) -> (268.5052, -434.1296)
  line L319 (268.5052, -434.1296) -> (268.5052, -413.8472)
  line L320 (268.5052, -413.8472) -> (264.7997, -413.8472)
  line L321 (264.7997, -413.8472) -> (264.7997, -393.9649)
  line L322 (264.7997, -393.9649) -> (268.5052, -393.9649)
  line L323 (268.5052, -393.9649) -> (268.5052, -373.6825)
  line L324 (-244.5787, -21.5839) -> (-244.5787, -327.7839)
  line L325 (-244.5787, -327.7839) -> (-235.912, -327.7839)
  line L326 (-235.912, -327.7839) -> (-235.912, -331.7839)
  line L327 (-235.912, -331.7839) -> (-227.0454, -331.7839)
  line L328 (-227.0454, -331.7839) -> (-227.0454, -327.7839)
  line L329 (-227.0454, -327.7839) -> (-218.3787, -327.7839)
  line L330 (-218.3787, -327.7839) -> (-218.3787, -303.2384)
  line L331 (-218.3787, -303.2384) -> (-214.3787, -303.2384)
  line L332 (-214.3787, -303.2384) -> (-214.3787, -274.4929)
  line L333 (-214.3787, -274.4929) -> (-218.3787, -274.4929)
  line L334 (-218.3787, -274.4929) -> (-218.3787, -246.1475)
  line L335 (-218.3787, -246.1475) -> (-214.3787, -246.1475)
  line L336 (-214.3787, -246.1475) -> (-214.3787, -217.402)
  line L337 (-214.3787, -217.402) -> (-218.3787, -217.402)
  line L338 (-218.3787, -217.402) -> (-218.3787, -189.0566)
  line L339 (-218.3787, -189.0566) -> (-214.3787, -189.0566)
  line L340 (-214.3787, -189.0566) -> (-214.3787, -160.3111)
  line L341 (-214.3787, -160.3111) -> (-218.3787, -160.3111)
  line L342 (-218.3787, -160.3111) -> (-218.3787, -131.9657)
  line L343 (-218.3787, -131.9657) -> (-214.3787, -131.9657)
  line L344 (-214.3787, -131.9657) -> (-214.3787, -103.2202)
  line L345 (-214.3787, -103.2202) -> (-218.3787, -103.2202)
  line L346 (-218.3787, -103.2202) -> (-218.3787, -74.8748)
  line L347 (-218.3787, -74.8748) -> (-214.3787, -74.8748)
  line L348 (-214.3787, -74.8748) -> (-214.3787, -46.1293)
  line L349 (-214.3787, -46.1293) -> (-218.3787, -46.1293)
  line L350 (-218.3787, -46.1293) -> (-218.3787, -21.5839)
  line L351 (-218.3787, -21.5839) -> (-227.0454, -21.5839)
  line L352 (-227.0454, -21.5839) -> (-227.0454, -17.5839)
  line L353 (-227.0454, -17.5839) -> (-235.912, -17.5838)
  line L354 (-235.912, -17.5838) -> (-235.912, -21.5839)
  line L355 (-235.912, -21.5839) -> (-244.5787, -21.5839)
  line L356 (398.8717, -302.2996) -> (398.8717, -322.1996)
  line L357 (398.8717, -322.1996) -> (394.8717, -322.1996)
  line L358 (394.8717, -322.1996) -> (394.8717, -342.3996)
  line L359 (394.8717, -342.3996) -> (398.8717, -342.3996)
  line L360 (398.8717, -342.3996) -> (398.8717, -362.1996)
  line L361 (398.8717, -362.1996) -> (394.8717, -362.1996)
  line L362 (394.8717, -362.1996) -> (394.8717, -382.3996)
  line L363 (394.8717, -382.3996) -> (398.8717, -382.3996)
  line L364 (398.8717, -382.3996) -> (398.8717, -402.1996)
  line L365 (398.8717, -402.1996) -> (394.8717, -402.1996)
  line L366 (394.8717, -402.1996) -> (394.8717, -422.3996)
  line L367 (394.8717, -422.3996) -> (423.6172, -422.3996)
  line L368 (423.6172, -422.3996) -> (423.6172, -418.3996)
  line L369 (423.6172, -418.3996) -> (451.9626, -418.3996)
  line L370 (451.9626, -418.3996) -> (451.9626, -422.3996)
  line L371 (451.9626, -422.3996) -> (480.7081, -422.3996)
  line L372 (480.7081, -422.3996) -> (480.7081, -418.3996)
  line L373 (480.7081, -418.3996) -> (509.0535, -418.3996)
  line L374 (509.0535, -418.3996) -> (509.0535, -422.3996)
  line L375 (509.0535, -422.3996) -> (537.799, -422.3996)
  line L376 (537.799, -422.3996) -> (537.799, -418.3996)
  line L377 (537.799, -418.3996) -> (566.1444, -418.3996)
  line L378 (566.1444, -418.3996) -> (566.1444, -422.3996)
  line L379 (566.1444, -422.3996) -> (594.8899, -422.3996)
  line L380 (594.8899, -422.3996) -> (594.8899, -418.3996)
  line L381 (594.8899, -418.3996) -> (623.2353, -418.3996)
  line L382 (623.2353, -418.3996) -> (623.2353, -422.3996)
  line L383 (623.2353, -422.3996) -> (651.9808, -422.3996)
  line L384 (651.9808, -422.3996) -> (651.9808, -418.3996)
  line L385 (651.9808, -418.3996) -> (680.3263, -418.3996)
  line L386 (680.3263, -418.3996) -> (680.3263, -422.3996)
  line L387 (680.3263, -422.3996) -> (709.0717, -422.3996)
  line L388 (709.0717, -422.3996) -> (709.0717, -402.1996)
  line L389 (709.0717, -402.1996) -> (705.0717, -402.1996)
  line L390 (705.0717, -402.1996) -> (705.0717, -382.3996)
  line L391 (705.0717, -382.3996) -> (709.0717, -382.3996)
  line L392 (709.0717, -382.3996) -> (709.0717, -362.1996)
  line L393 (709.0717, -362.1996) -> (705.0717, -362.1996)
  line L394 (705.0717, -362.1996) -> (705.0717, -342.3996)
  line L395 (705.0717, -342.3996) -> (709.0717, -342.3996)
  line L396 (709.0717, -342.3996) -> (709.0717, -322.1996)
  line L397 (709.0717, -322.1996) -> (705.0717, -322.1996)
  line L398 (705.0717, -322.1996) -> (705.0717, -302.3996)
  line L399 (705.0717, -302.3996) -> (709.0717, -302.3996)
  line L400 (709.0717, -302.3996) -> (709.0717, -282.1996)
  line L401 (709.0717, -282.1996) -> (705.0717, -282.1996)
  line L402 (705.0717, -282.1996) -> (705.0717, -262.3996)
  line L403 (705.0717, -262.3996) -> (709.0717, -262.3996)
  line L404 (709.0717, -262.3996) -> (709.0717, -242.1996)
  line L405 (709.0717, -242.1996) -> (705.0717, -242.1996)
  line L406 (705.0717, -242.1996) -> (705.0717, -222.3996)
  line L407 (705.0717, -222.3996) -> (709.0717, -222.3996)
  line L408 (709.0717, -222.3996) -> (709.0717, -202.1996)
  line L409 (709.0717, -202.1996) -> (394.8717, -202.1996)
  line L410 (394.8717, -202.1996) -> (394.8717, -222.3996)
  line L411 (394.8717, -222.3996) -> (398.8717, -222.3996)
  line L412 (398.8717, -222.3996) -> (398.8717, -242.1996)
  line L413 (398.8717, -242.1996) -> (394.8717, -242.1996)
  line L414 (394.8717, -242.1996) -> (394.8717, -262.3996)
  line L415 (394.8717, -262.3996) -> (398.8717, -262.3996)
  line L416 (398.8717, -262.3996) -> (398.8717, -282.1996)
  line L417 (398.8717, -282.1996) -> (394.8717, -282.1996)
  line L418 (394.8717, -282.1996) -> (394.8717, -302.2996)
  line L419 (350.1751, -274.0319) -> (358.1749, -274.0349)
  line L420 (358.1749, -274.0349) -> (358.1818, -253.7525)
  line L421 (358.1818, -253.7525) -> (350.1821, -253.7496)
  line L422 (350.1821, -253.7496) -> (350.1889, -233.8672)
  line L423 (350.1889, -233.8672) -> (358.1887, -233.8702)
  line L424 (358.1887, -233.8702) -> (358.1956, -213.5784)
  line L425 (358.1956, -213.5784) -> (312.1759, -217.7448)
  line L426 (312.1759, -217.7448) -> (313.9797, -237.6632)
  line L427 (313.9797, -237.6632) -> (309.9961, -238.0239)
  line L428 (309.9961, -238.0239) -> (311.818, -258.1414)
  line L429 (311.818, -258.1414) -> (315.8016, -257.7808)
  line L430 (315.8016, -257.7808) -> (317.5874, -277.5)
  line L431 (317.5874, -277.5) -> (313.6038, -277.8607)
  line L432 (313.6038, -277.8607) -> (315.4257, -297.9782)
  line L433 (315.4257, -297.9782) -> (319.4092, -297.6176)
  line L434 (319.4092, -297.6176) -> (321.195, -317.3368)
  line L435 (321.195, -317.3368) -> (317.2114, -317.6974)
  line L436 (317.2114, -317.6974) -> (319.0333, -337.815)
  line L437 (319.0333, -337.815) -> (323.0169, -337.4544)
  line L438 (323.0169, -337.4544) -> (324.8027, -357.1736)
  line L439 (324.8027, -357.1736) -> (320.8191, -357.5342)
  line L440 (320.8191, -357.5342) -> (322.641, -377.6518)
  line L441 (322.641, -377.6518) -> (326.6245, -377.2912)
  line L442 (326.6245, -377.2912) -> (328.4103, -397.0104)
  line L443 (328.4103, -397.0104) -> (324.4267, -397.371)
  line L444 (324.4267, -397.371) -> (326.2486, -417.4886)
  line L445 (326.2486, -417.4886) -> (330.2322, -417.128)
  line L446 (330.2322, -417.128) -> (332.036, -437.0464)
  line L447 (332.036, -437.0464) -> (340.8663, -436.2469)
  line L448 (340.8663, -436.2469) -> (340.5055, -432.2632)
  line L449 (340.5055, -432.2632) -> (348.9374, -431.4998)
  line L450 (348.9374, -431.4998) -> (349.2982, -435.4835)
  line L451 (349.2982, -435.4835) -> (358.1198, -434.6848)
  line L452 (358.1198, -434.6848) -> (358.1267, -414.4112)
  line L453 (358.1267, -414.4112) -> (350.127, -414.4082)
  line L454 (350.127, -414.4082) -> (350.1338, -394.5259)
  line L455 (350.1338, -394.5259) -> (358.1335, -394.5289)
  line L456 (358.1335, -394.5289) -> (358.1405, -374.2465)
  line L457 (358.1405, -374.2465) -> (350.1408, -374.2436)
  line L458 (350.1408, -374.2436) -> (350.1476, -354.3612)
  line L459 (350.1476, -354.3612) -> (358.1473, -354.3642)
  line L460 (358.1473, -354.3642) -> (358.1543, -334.0819)
  line L461 (358.1543, -334.0819) -> (350.1545, -334.0789)
  line L462 (350.1545, -334.0789) -> (350.1614, -314.1966)
  line L463 (350.1614, -314.1966) -> (358.1611, -314.1995)
  line L464 (358.1611, -314.1995) -> (358.1681, -293.9172)
  line L465 (358.1681, -293.9172) -> (350.1683, -293.9142)
  line L466 (350.1683, -293.9142) -> (350.1751, -274.0319)
  line L467 (224.5997, -406.7283) -> (4.7997, -406.7283)
  line L468 (4.7997, -406.7283) -> (4.7997, -286.929)
  line L469 (4.7997, -286.929) -> (224.5997, -286.929)
  line L470 (224.5997, -286.929) -> (224.5997, -406.7283)
  dimension "d85" = 0.1
hidden bodies 6 7 8 9 10
equation "lengd = 314 mm"
equation "hæð1 = 50 mm"
equation "hæð2 = 30 mm"
equation "breidd = 220 mm"
equation "þykkt = 4 mm"
equation "bfingur = 5"
equation "bfingurBreidd = breidd / ( ( bfingur * 2 ) + 1 )"
equation "d8 = lengd"
equation "d9 = breidd"
equation "d10 = þykkt"
equation "d12 = bfingurBreidd"
equation "d13 = bfingurBreidd"
equation "d14 = -þykkt"
equation "d16 = bfingur"
equation "d18 = breidd - bfingurBreidd * 3"
equation "d20 = hæð1"
equation "d21 = hæð2"
equation "d22 = þykkt"
equation "hfingur = 5"
equation "hbreidd = ( sqrt(( 50 - 30 ) ^ 2 + 220 ^ 2) ) * 1 mm"
equation "hfingurbreidd = hbreidd / ( hfingur * 2 + 1 )"
equation "d27 = hfingurbreidd"
equation "d28 = hfingurbreidd"
equation "d29 = -þykkt * 2"
equation "d31 = hfingur"
equation "d33 = hbreidd - hfingurbreidd * 3"
equation "lfingur = 5"
equation "lfingurbreidd = lengd / ( lfingur * 2 + 1 )"
equation "d42 = lfingurbreidd"
equation "d43 = lfingurbreidd"
equation "d44 = -þykkt"
equation "d46 = lfingur"
equation "d48 = -( lengd - lfingurbreidd * 3 )"
equation "hliðarfingurframanbreidd = ( hæð2 - þykkt ) / ( hliðarfingurframan * 2 + 1 )"
equation "hliðarfingurframan = 1"
equation "d56 = hliðarfingurframanbreidd"
equation "d57 = hliðarfingurframanbreidd"
equation "d58 = -þykkt"
equation "d61 = -þykkt"
equation "haldaribreidd = 50 mm"
equation "halfurkerf = 0.1 mm"
equation "d75 = þykkt"
equation "d77 = -þykkt"
equation "miðjubillengd = 220 mm"
equation "miðjubilhæð = 120 mm"
equation "d81 = miðjubillengd"
equation "d82 = miðjubilhæð"
equation "d83 = -þykkt"
equation "d85 = halfurkerf"
